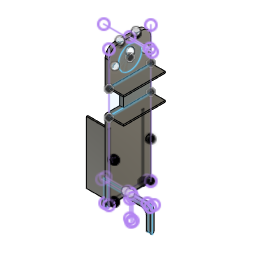
Body (Autodesk Fusion 360 design; units mm, degrees)
Autodesk Fusion 360 part; units mm, degrees
sketch "스케치1" plane through (0, 0, 0) normal (0, 1, 0) x (1, 0, 0)
  line L0 (-25, 0) -> (-25, -25)
  line L1 (-25, -25) -> (25, -25)
  line L2 (25, -25) -> (25, 0)
  line L3 (25, 0) -> (21, 0)
  line L4 (21, 0) -> (21, -21)
  line L5 (21, -21) -> (-21, -21)
  line L6 (-21, -21) -> (-21, 0)
  line L7 (-21, 0) -> (-25, 0)
  constraint vertical L0
  constraint perpendicular L0 L1
  constraint perpendicular L1 L2
  constraint perpendicular L2 L3
  constraint perpendicular L1 L4
  constraint perpendicular L0 L5
  constraint perpendicular L5 L6
  constraint perpendicular L0 L7
extrude "돌출1" add sketch "스케치1" along normal mid plane 4
sketch "스케치2" plane through (0, 0, 25) normal (0, 0, 1) x (-1, 0, 0)
  line L0 (25, 2) -> (-25, 2)
  line L1 (2, -21.65) -> (-2, -21.65)
  line L2 (2, -21.65) -> (2, 0)
  line L3 (-2, -21.65) -> (-2, 0)
  line L4 (-20, 0) -> (-2.5, 0)
  line L5 (2, 21.65) -> (-2, 21.65)
  line L6 (2, 21.65) -> (2, 0)
  line L7 (-2, 21.65) -> (-2, 0)
  line L8 (25, -2) -> (-25, -2)
  dimension "d29" = 21.65
  dimension "d30" = 2
  dimension "d31" = 2
  constraint perpendicular L1 L2
  constraint perpendicular L1 L3
  constraint symmetric L1.start L4 L5.start
  constraint symmetric L1.end L4 L5.end
  constraint symmetric L2.end L4 L6.end
  constraint symmetric L3.end L4 L7.end
  measures "d29" distance of L1 L4
  measures "d30" distance of L2 origin
  measures "d31" distance of origin L3
extrude "돌출2" add sketch "스케치2" along normal blind 140
sketch "스케치14" plane through (0, 0, 165) normal (0, 0, 1) x (-1, 0, 0)
  circle A0 centre (0, -8.4) radius 1.8
  line L0 (-1.75, 0) -> (-22.5, 0)
  circle A1 centre (0, 8.4) radius 1.8
  dimension "d34" = 3.6
  dimension "d35" = 8.4
  constraint symmetric A0 L0 A1
  measures "d34" diameter of A0
  measures "d35" distance of A0.centre L0
extrude "돌출10" cut sketch "스케치14" against normal blind 1.87
sketch "스케치23" plane through (0, 0, 163.13) normal (0, 0, 1) x (-1, 0, 0)
  circle A0 centre (0, -8.4) radius 1.25
  line L0 (25, 0) -> (-25, 0)
  circle A1 centre (0, 8.4) radius 1.25
  point P0 (0, -8.4)
  dimension "d96" = 2.5
  constraint coincident P0 A0.centre
  constraint symmetric A0 L0 A1
  measures "d96" diameter of A0
extrude "돌출22" cut sketch "스케치23" against normal blind 3
sketch "스케치15" plane through (2, 0, 0) normal (1, 0, 0) x (0, 1, 0)
  line L0 (0, 1.75) -> (0, 22.5)
  line L1 (-21.65, 165) -> (21.65, 165)
  circle A0 centre (-18.85, 27.8) radius 2.5
  line L2 (2, 25) -> (21.65, 25)
  line L3 (-21.65, 25) -> (-21.65, 165)
  circle A1 centre (-18.85, 65.5) radius 2.5
  circle A2 centre (18.85, 65.5) radius 2.5
  circle A3 centre (18.85, 27.8) radius 2.5
  dimension "d43" = 5
  dimension "d44" = 2.8
  dimension "d45" = 2.8
  dimension "d46" = 5
  dimension "d47" = 37.7
  constraint symmetric L0 A0 A3
  constraint symmetric L0 A1 A2
  measures "d43" diameter of A0
  measures "d44" distance of A0.centre L2
  measures "d45" distance of A0.centre L3
  measures "d46" diameter of A1
  measures "d47" distance of A0.centre A1.centre
extrude "돌출13" add sketch "스케치15" along normal blind 3
sketch "스케치17" plane through (5, 0, 0) normal (1, 0, 0) x (0, 1, 0)
  circle A0 centre (-18.85, 65.5) radius 1.8
  circle A1 centre (-18.85, 27.8) radius 1.8
  line L0 (0, 1.75) -> (0, 22.5)
  circle A2 centre (18.85, 27.8) radius 1.8
  circle A3 centre (18.85, 65.5) radius 1.8
  point P0 (-18.85, 65.5)
  point P1 (-18.85, 27.8)
  dimension "d56" = 3.6
  dimension "d57" = 3.6
  constraint coincident P0 A0.centre
  constraint coincident P1 A1.centre
  constraint symmetric A0 L0 A3
  constraint symmetric A1 L0 A2
  measures "d56" diameter of A0
  measures "d57" diameter of A1
extrude "돌출15" cut sketch "스케치17" against normal blind 1.7
sketch "스케치21" plane through (3.3, 0, 0) normal (1, 0, 0) x (0, 1, 0)
  circle A0 centre (-18.85, 65.5) radius 1.25
  circle A1 centre (-18.85, 27.8) radius 1.25
  line L0 (0, 25) -> (0, 0)
  circle A2 centre (18.85, 65.5) radius 1.25
  point P0 (-18.85, 65.5)
  point P1 (-18.85, 27.8)
  point P2 (18.85, 27.8)
  dimension "d89" = 2.5
  dimension "d90" = 2.5
  constraint coincident P0 A0.centre
  constraint coincident P1 A1.centre
  constraint symmetric A0 L0 A2
  constraint symmetric P1 L0 P2
  measures "d89" diameter of A0
  measures "d90" diameter of A1
extrude "돌출20" cut sketch "스케치21" 1 faces at (3.3, 18.6189, 27.6425) against normal blind 3
sketch "스케치18" plane through (2, 0, 0) normal (1, 0, 0) x (0, 1, 0)
  line L0 (-21.65, 103.4083) -> (21.65, 103.4083)
  line L1 (21.65, 103.4083) -> (21.65, 104.9083)
  line L2 (21.65, 104.9083) -> (-21.65, 104.9083)
  line L3 (-21.65, 104.9083) -> (-21.65, 103.4083)
  line L4 (-21.65, 25) -> (-21.65, 165)
  line L5 (21.65, 25) -> (21.65, 165)
  line L6 (-21.65, 129.4083) -> (21.65, 129.4083)
  line L7 (21.65, 129.4083) -> (21.65, 130.9083)
  line L8 (21.65, 130.9083) -> (-21.65, 130.9083)
  line L9 (-21.65, 130.9083) -> (-21.65, 129.4083)
  dimension "d60" = 1.5
  dimension "d61" = 1.5
  dimension "d62" = 24.5
  constraint horizontal L0
  constraint vertical L1
  constraint horizontal L2
  constraint vertical L3
  constraint coincident L1.end L5
  constraint coincident L0.start L4
  constraint horizontal L6
  constraint vertical L7
  constraint horizontal L8
  constraint vertical L9
  constraint coincident L5 L7.end
  constraint coincident L4 L6.start
  measures "d60" distance of L0.end L1.end
  measures "d61" distance of L6.end L7.end
  measures "d62" distance of L1.end L6.end
extrude "돌출16" add sketch "스케치18" along normal blind 15 contours L0 L1 L2 L3 L4 L5 | L4 L5 L6 L7 L8 L9
sketch "스케치19" plane through (2, 0, 0) normal (1, 0, 0) x (0, 1, 0)
  circle A0 centre (0, 146.9177) radius 12
  circle A1 centre (15.7, 146.9177) radius 1.8
  line L0 (0, 2.5) -> (0, 20)
  circle A2 centre (-15.7, 146.9177) radius 1.8
  circle A3 centre (0, 152.4177) radius 3.5
  circle A4 centre (0, 152.4177) radius 1.8
  dimension "d65" = 24
  dimension "d66" = 3.6
  dimension "d67" = 15.7
  dimension "d68" = 7
  dimension "d69" = 5.5
  dimension "d70" = 3.6
  constraint symmetric A1 L0 A2
  constraint concentric A3 A4
  constraint coincident A0.centre L0
  measures "d65" diameter of A0
  measures "d66" diameter of A1
  measures "d67" distance of A0.centre A1.centre
  measures "d68" diameter of A3
  measures "d69" distance of A0.centre A3.centre
  measures "d70" diameter of A4
extrude "돌출17" cut sketch "스케치19" against normal blind 1.7 contours A1 | A2
sketch "스케치22" plane through (0.3, 0, 0) normal (1, 0, 0) x (0, 1, 0)
  circle A0 centre (-15.7, 146.9177) radius 1.25
  line L0 (0, 25) -> (0, 0)
  circle A1 centre (15.7, 146.9177) radius 1.25
  point P0 (-15.7, 146.9177)
  dimension "d93" = 2.5
  constraint coincident P0 A0.centre
  constraint symmetric A0 L0 A1
  measures "d93" diameter of A0
extrude "돌출21" cut sketch "스케치22" against normal blind 2
extrude "돌출18" cut sketch "스케치19" against normal through all contours A3 | A4
sketch "스케치20" plane through (-2, 0, 0) normal (-1, 0, 0) x (0, -1, 0)
  line L0 (-2, 25) -> (-21.65, 25)
  line L1 (-16.65, 25) -> (-16.65, 89.5)
  line L2 (16.65, 25) -> (16.65, 89.5)
  line L3 (-16.65, 89.5) -> (-18.15, 89.5)
  line L4 (-18.15, 89.5) -> (-18.15, 25)
  line L5 (-18.15, 25) -> (-16.65, 25)
  line L6 (16.65, 25) -> (18.15, 25)
  line L7 (18.15, 25) -> (18.15, 89.5)
  line L8 (18.15, 89.5) -> (16.65, 89.5)
  point P0 (21.65, 25)
  dimension "d74" = 33.3
  dimension "d75" = 5
  dimension "d76" = 5
  dimension "d77" = 1.5
  dimension "d78" = 1.5
  dimension "d79" = 64.5
  constraint coincident L0 L1.start
  constraint perpendicular L0 L1
  constraint vertical L2
  constraint perpendicular L1 L3
  constraint coincident L0 L4.end
  constraint perpendicular L0 L4
  constraint perpendicular L2 L6
  constraint perpendicular L6 L7
  constraint perpendicular L2 L8
  measures "d74" distance of L1.end L2.end
  measures "d75" distance of L2.start P0
  measures "d76" distance of L0.end L1.start
  measures "d77" distance of L1.end L3.end
  measures "d78" distance of L2.start L6.end
  measures "d79" distance of L3.end L4.end
extrude "돌출19" add sketch "스케치20" along normal blind 23
fillet "모깎기1" radius 5 4 edges at (-21, 0, 21) (-25, 0, 25) (21, 0, 21) (25, 0, 25)
fillet "모깎기2" radius 2 4 edges at (-23, -2, 0) (-23, 2, 0) (23, -2, 0) (23, 2, 0)
fillet "모깎기3" radius 5 2 edges at (0, -2, 25) (0, 2, 25)
sketch "스케치24" plane through (-2, 0, 0) normal (-1, 0, 0) x (0, -1, 0)
  line L0 (-21.65, 129.4083) -> (21.65, 129.4083)
  line L1 (21.65, 130.9083) -> (21.65, 129.4083)
  line L2 (21.65, 129.4083) -> (6.65, 129.4083)
  line L3 (21.65, 104.9083) -> (-21.65, 104.9083)
  line L4 (6.65, 129.4083) -> (6.65, 104.9083)
  line L5 (6.65, 104.9083) -> (21.65, 104.9083)
  line L6 (21.65, 104.9083) -> (21.65, 129.4083)
  point P0 (21.65, 129.4083)
  dimension "d99" = 15
  constraint coincident P0 L0.end
  constraint coincident L0 L2.end
  constraint coincident L3 L4.end
  constraint perpendicular L2 L4
  constraint coincident L3.start L5.end
  measures "d99" distance of P0 L2.end
extrude "돌출23" cut sketch "스케치24" against normal through all
fillet "모깎기4" radius 10 2 edges at (0, 21.65, 165) (0, -21.65, 165)
equation "d35 = 10 mm - 1.6 mm"
equation "d67 = 18.5 mm - 2.8 mm"
equation "d69 = 8.5 mm - 3 mm"
